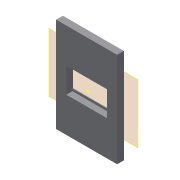
# Autodesk Inventor part: 03_MountCoverslip
Saved by Autodesk Inventor 2019.4 (Build 234330000, 330)
## iProperties
Created: 2020-11-17
Part Number: 03_MountCoverslip
Material: Generic
Document SubType Name: Modeling
Designer: diederichbenedict
Density: 1 g/cm^3
Appearance: Default
Author: diederichbenedict
Autodesk Inventor part; units mm, degrees
ref_plane "YZ Plane" through (0, 0, 0) normal (1, 0, 0) x (0, 1, 0)
ref_plane "XZ Plane" through (0, 0, 0) normal (0, 1, 0) x (-1, 0, 0)
ref_plane "XY Plane" through (0, 0, 0) normal (0, 0, 1) x (1, 0, 0)
ref_plane "Work Plane1" through (0, 0, 0) normal (0, 0, 1) x (1, 0, 0)
sketch "Sketch1" plane through (0, 0, 0) normal (0, 0, 1) x (1, 0, 0)
  circle A0 centre (15, 28) radius 2.45 projected
  circle A1 centre (-15, 28) radius 2.45 projected
  circle A2 centre (0, -26.0002) radius 2.45 projected
  line L0 (-22.5, -35) -> (22.5, -35)
  line L1 (22.5, -35) -> (22.5, 35)
  line L2 (22.5, 35) -> (-22.5, 35)
  line L3 (-22.5, 35) -> (-22.5, -35)
  line L4 (-22.5, -35) -> (22.5, 35) construction
  line L5 (22.5, -35) -> (-22.5, 35) construction
  line L6 (-15, -7.5) -> (15, -7.5)
  line L7 (15, -7.5) -> (15, 7.5)
  line L8 (15, 7.5) -> (-15, 7.5)
  line L9 (-15, 7.5) -> (-15, -7.5)
  line L10 (-15, -7.5) -> (15, 7.5) construction
  line L11 (15, -7.5) -> (-15, 7.5) construction
  point P0 (0, 0)
  dimension "d0" = 45
  dimension "d1" = 70
  dimension "d2" = 30
  dimension "d3" = 15
  constraints: 24 end point, 4 midpoint, 4 parallel, 2 horizontal, 2 perpendicular
  measures "d0" distance of L2.end L1.end
  measures "d1" distance of L1.end L0.end
  measures "d2" distance of L8.end L7.end
  measures "d3" distance of L7.end L6.end
extrude "Extrusion1" add sketch "Sketch1" along normal blind 4
sketch "Sketch2" plane through (0, 0, 4) normal (0, 0, 1) x (1, 0, 0)
  point P0 (0, 0)
sketch "Sketch3" plane through (0, 0, 4) normal (0, 0, 1) x (1, 0, 0)
  line L0 (-15, -7.5) -> (-15, 7.5) projected
  line L1 (-15, 7.5) -> (15, 7.5) projected
  line L2 (15, 7.5) -> (15, -7.5) projected
  line L3 (15, -7.5) -> (-15, -7.5) projected
  circle A0 centre (0, -26.0002) radius 2.45 projected
  circle A1 centre (-15, 28) radius 2.45 projected
  circle A2 centre (15, 28) radius 2.45 projected
  line L4 (-22.5, -35) -> (22.5, -35) projected
  line L5 (22.5, -35) -> (22.5, 35) projected
  line L6 (22.5, 35) -> (-22.5, 35) projected
  line L7 (-22.5, 35) -> (-22.5, -35) projected
  point P0 (0, 0)
extrude "Extrusion2" add sketch "Sketch3" along normal blind 1 contours A0 | A1 | A2 | L7 L6 L5 L4
sketch "Sketch4" plane through (0, 0, 5) normal (0, 0, 1) x (1, 0, 0)
  line L0 (-15, -9.25) -> (15, -9.25)
  line L1 (15, -9.25) -> (15, 9.25)
  line L2 (15, 9.25) -> (-15, 9.25)
  line L3 (-15, 9.25) -> (-15, -9.25)
  line L4 (-15, -9.25) -> (15, 9.25) construction
  line L5 (15, -9.25) -> (-15, 9.25) construction
  point P0 (0, 0)
  dimension "d8" = 30
  dimension "d9" = 18.5
  constraints: 12 end point, 2 midpoint, 2 parallel, 1 horizontal, 1 perpendicular
  measures "d8" distance of L2.end L1.end
  measures "d9" distance of L1.end L0.end
extrude "Extrusion3" cut sketch "Sketch4" against normal blind 4.5
body "Solid1"
